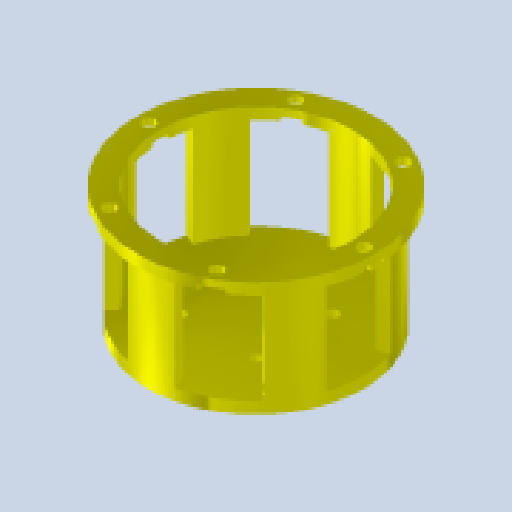
# Autodesk Inventor part: Soporte_Motor
Saved by Autodesk Inventor 2025.3 (Build 293356030, 356C)
## iProperties
Created: 2025-10-12
Part Number: Soporte_Motor
Material: Aluminio 7075
Document SubType Name: Modeling
Designer: santa
Density: 2.81 g/cm^3
Appearance: Anodizado - Azul
Author: santa
Autodesk Inventor part; units mm, degrees
ref_plane "YZ Plane" through (0, 0, 0) normal (1, 0, 0) x (0, 1, 0)
ref_plane "XZ Plane" through (0, 0, 0) normal (0, 1, 0) x (-1, 0, 0)
ref_plane "XY Plane" through (0, 0, 0) normal (0, 0, 1) x (1, 0, 0)
sketch "Boceto1" plane through (0, 0, 0) normal (0, 0, 1) x (1, 0, 0)
  circle A0 centre (0, 0) radius 25
  line L0 (-10, 10) -> (10, 10) construction
  line L1 (10, 10) -> (10, -10) construction
  line L2 (10, -10) -> (-10, -10) construction
  line L3 (-10, -10) -> (-10, 10) construction
  line L4 (-10, 10) -> (10, -10) construction
  line L5 (10, 10) -> (-10, -10) construction
  circle A1 centre (0, 0) radius 28
  line L6 (0, 0) -> (-24.4074, -5.411) construction
  line L7 (0, 0) -> (-24.4074, 5.411) construction
  line L8 (-28, 0) -> (0, 0)
  line L9 (-24.4074, -5.411) -> (-27.3363, -6.0603)
  line L10 (-24.4074, 5.411) -> (-27.3363, 6.0603)
  line L11 (-7.5176, -23.8429) -> (-8.4198, -26.7041)
  line L12 (-16.8898, -18.4319) -> (-18.9165, -20.6438)
  line L13 (16.8898, -18.4319) -> (18.9165, -20.6438)
  line L14 (7.5176, -23.8429) -> (8.4198, -26.7041)
  line L15 (24.4074, 5.411) -> (27.3363, 6.0603)
  line L16 (24.4074, -5.411) -> (27.3363, -6.0603)
  line L17 (7.5176, 23.8429) -> (8.4198, 26.7041)
  line L18 (16.8898, 18.4319) -> (18.9165, 20.6438)
  line L19 (-16.8898, 18.4319) -> (-18.9165, 20.6438)
  line L20 (-7.5176, 23.8429) -> (-8.4198, 26.7041)
  point P0 (7.5176, -23.8429)
  point P1 (8.4198, -26.7041)
  point P2 (16.8898, -18.4319)
  point P3 (24.4074, -5.411)
  point P4 (27.3363, -6.0603)
  point P5 (27.3363, 6.0603)
  point P6 (24.4074, 5.411)
  point P7 (16.8898, 18.4319)
  point P8 (18.9165, 20.6438)
  point P9 (8.4198, 26.7041)
  point P10 (-7.5176, 23.8429)
  point P11 (-8.4198, 26.7041)
  point P12 (-18.9165, 20.6438)
  point P13 (-16.8898, -18.4319)
  point P14 (-18.9165, -20.6438)
  dimension "d0" = 50
  dimension "d1" = 20
  dimension "d2" = 56
  dimension "d7" = 25
  dimension "d10" = 360
  constraints: 42 end point, 6 coincident, 5 point on circle, 2 centre point, 2 collinear, 2 horizontal, 2 midpoint, 2 parallel, 2 perpendicular, 38 other
  measures "d0" diameter of A0
  measures "d1" distance of L1.end L2.end
  measures "d2" diameter of A1
  measures "d7" angle of L6 L7
extrude "Extrusión1" add sketch "Boceto1" along normal blind 3 contours A0 | A0 L18 A1 L15 | L16 A1 L13 A0 | A0 L20 A1 L17 | L14 A1 L11 A0 | A0 L10 A1 L19 | L12 A1 L9 A0
extrude "Extrusión2" add sketch "Boceto1" along normal blind 32 contours A0 L15 A1 L16 | A0 L17 A1 L18 | L13 A1 L14 A0 | A0 L19 A1 L20 | L11 A1 L12 A0 | A0 L8 A1 L10 | L9 A1 L8 A0
ref_plane "Plano de trabajo1" through (0, 0, 32) normal (0, 0, -1) x (-1, 0, 0)
sketch "Boceto2" plane through (0, 0, 32) normal (0, 0, -1) x (-1, 0, 0)
  circle A0 centre (0, 0) radius 25 projected
  circle A1 centre (0, 0) radius 28 projected
  circle A2 centre (0, 0) radius 31
  arc A3 (18.9165, 20.6438) -> (8.4198, 26.7041) centre (0, 0) ccw projected
  line L0 (18.9165, 20.6438) -> (16.8898, 18.4319) projected
  arc A4 (16.8898, 18.4319) -> (7.5176, 23.8429) centre (0, 0) ccw projected
  line L1 (7.5176, 23.8429) -> (8.4198, 26.7041) projected
  arc A5 (27.3363, -6.0603) -> (27.3363, 6.0603) centre (0, 0) ccw projected
  line L2 (27.3363, -6.0603) -> (24.4074, -5.411) projected
  arc A6 (24.4074, -5.411) -> (24.4074, 5.411) centre (0, 0) ccw projected
  line L3 (24.4074, 5.411) -> (27.3363, 6.0603) projected
  line L4 (0, 0) -> (26.8468, 15.5) construction
  point P0 (24.2487, 14)
  point P1 (0, 28)
  point P2 (-24.2487, 14)
  point P3 (-24.2487, -14)
  point P4 (0, -28)
  point P5 (24.2487, -14)
  dimension "d13" = 3
  dimension "d16" = 17.5
  dimension "d19" = 360
  constraints: 2 end point, 1 point on line, 12 other
  measures "d16" angle of L3 L4
extrude "Extrusión3" add sketch "Boceto2" along normal blind 3 contours A0 L3 A1 L2 | A0 L0 A1 L3 | L2 A1 L1 A0 | A0 L1 A1 L0 | A2
hole "Agujero1" at (-24.2487, 14, 32) at (-24.2487, -14, 32) at (0, 28, 32) at (24.2487, 14, 32) at (24.2487, -14, 32) at (0, -28, 32) direction (0, 0, -1) diameter 3.4 depth 3 clearance for "Tornillo de cabeza hueca" size "M3" standard "Perfil M métrico ANSI"
hole "Agujero2" at (10, 10, 0) at (10, -10, 0) at (-10, -10, 0) at (-10, 10, 0) direction (0, 0, 1) diameter 2.9 end through all clearance for "Tornillo de cabeza hueca" size "M2.5" standard "Perfil M métrico ANSI"
sketch "Boceto3" plane through (0, 0, 29) normal (0, 0, -1) x (-1, 0, 0)
  circle A0 centre (24.2487, 14) radius 1.6 projected
  circle A1 centre (24.2487, 14) radius 3.2
  circle A2 centre (24.2487, 14) radius 4
  point P0 (0, 0)
  dimension "d35" = 6.4
  dimension "d45" = 8
  constraints: 2 centre point, 2 coincident
  measures "d35" diameter of A1
  measures "d45" diameter of A2
extrude "Extrusión4" cut sketch "Boceto3" against normal blind 1 contours A1
extrude "Extrusión5" cut sketch "Boceto3" along normal through all contours A0 | A1 | A2
fillet "Empalme1" radius 0.5 4 edges at (-26.2419, 16.5035, 29.5) (-27.4134, 14.4744, 29.5) (-21.1055, 13.4, 29.5) (-22.1574, 11.5779, 29.5)
fillet "Empalme1" radius 2 2 edges at (-22.0064, 17.3124, 1.5) (-25.9962, 10.4019, 1.5)
pattern_circular "Patrón circular1" count 6 over 360 about axis through (0, 0, 0) along (0, 0, 1) of "Empalme1", "Extrusión4", "Extrusión5"
equation "\"d12\" = -d5"
equation "\"d5\" = 32"
